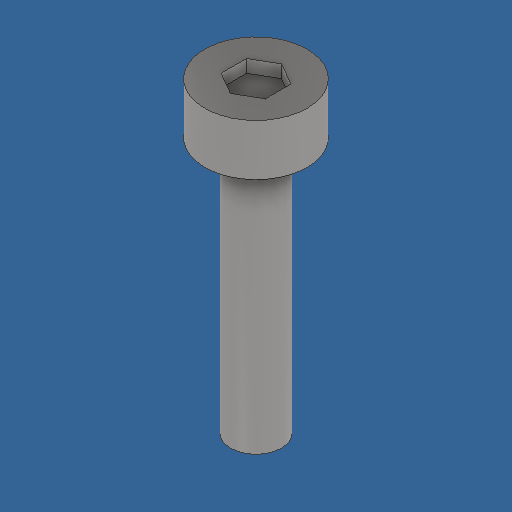
# Autodesk Inventor part: 4mm_screw
Saved by Autodesk Inventor 2026.2 (Build 302298000, 298)
## iProperties
Created: 2026-01-15
Part Number: 4mm_screw
Material: Stainless Steel
Document SubType Name: Modeling
Designer: Thoma
Density: 8 g/cm^3
Appearance: Semi-Polished
Author: Thoma
Autodesk Inventor part; units mm, degrees
ref_plane "YZ Plane" through (0, 0, 0) normal (1, 0, 0) x (0, 1, 0)
ref_plane "XZ Plane" through (0, 0, 0) normal (0, 1, 0) x (-1, 0, 0)
ref_plane "XY Plane" through (0, 0, 0) normal (0, 0, 1) x (1, 0, 0)
sketch "Sketch1" plane through (0, 0, 0) normal (0, 1, 0) x (-1, 0, 0)
  circle A0 centre (0, 0) radius 2.5
  circle A1 centre (0, 0) radius 1
  dimension "d0" = 5
  constraints: 2 centre point, 2 coincident
  measures "d0" diameter of A0
extrude "Extrusion1" add sketch "Sketch1" against normal blind 10 contours A1
sketch "Sketch2" plane through (0, 0, 0) normal (0, 1, 0) x (1, 0, 0)
  circle A0 centre (0, 0) radius 2
  dimension "d3" = 4
  constraints: 1 centre point, 1 coincident
  measures "d3" diameter of A0
extrude "Extrusion2" add sketch "Sketch2" along normal blind 2
sketch "Sketch3" plane through (0, 2, 0) normal (0, 1, 0) x (1, 0, 0)
  circle A0 centre (0, 0) radius 1 projected
  line L0 (0, 1) -> (0.866, 0.5)
  line L1 (0.866, 0.5) -> (0.866, -0.5)
  line L2 (0.866, -0.5) -> (0, -1)
  line L3 (0, -1) -> (-0.866, -0.5)
  line L4 (-0.866, -0.5) -> (-0.866, 0.5)
  line L5 (-0.866, 0.5) -> (0, 1)
  constraints: 12 end point, 1 coincident, 1 vertical alignment, 14 other
extrude "Extrusion3" cut sketch "Sketch3" against normal blind 0.5 contours L1 L2 L3 L4 L5 L0
body "Solid1"
